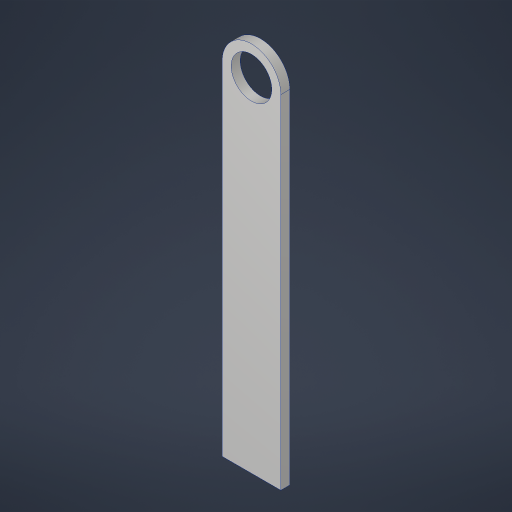
# Autodesk Inventor part: CL2-001
Saved by Autodesk Inventor 2023.4 (Build 274418000, 418)
## iProperties
Created: 2025-01-26
Part Number: CL2-001
Material: Aluminum 6061
Document SubType Name: Modeling
Designer: brand
Density: 2.7 g/cm^3
Appearance: Aluminum - Flat
Author: brand
Autodesk Inventor part; units mm, degrees
ref_plane "YZ Plane" through (0, 0, 0) normal (1, 0, 0) x (0, 1, 0)
ref_plane "XZ Plane" through (0, 0, 0) normal (0, 1, 0) x (-1, 0, 0)
ref_plane "XY Plane" through (0, 0, 0) normal (0, 0, 1) x (1, 0, 0)
sketch "Sketch1" plane through (0, 0, 0) normal (0, 0, 1) x (1, 0, 0)
  circle A0 centre (0, 0) radius 14.2875
  circle A1 centre (0, 0) radius 20.6375
  line L0 (20.6375, -241.3) -> (-20.6375, -241.3)
  line L1 (-20.6375, 0) -> (-20.6375, -241.3)
  line L2 (20.6375, -241.3) -> (20.6375, 0)
  dimension "d0" = 28.575
  dimension "d1" = 6.35
  dimension "d2" = 241.3
  constraints: 6 end point, 2 centre point, 2 point on circle, 2 tangent, 2 vertical, 1 coincident, 1 horizontal
  measures "d0" diameter of A0
  measures "d1" radial gap between concentric circles of A0 A1
  measures "d2" distance from line of L0 point (0, 0)
extrude "Extrusion1" add sketch "Sketch1" along normal mid plane 6.35
body "Solid1"
